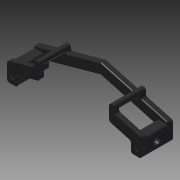
# Autodesk Inventor part: Solenoid Mount
Saved by Autodesk Inventor 2015 (Build 190159000, 159)
## iProperties
Created: 2016-09-23
Part Number: Solenoid Mount
Material: Generic
Document SubType Name: Modeling
Designer: James Yelland
Density: 1 g/cm^3
Appearance: Default
Author: James Yelland
Autodesk Inventor part; units mm, degrees
ref_plane "YZ Plane" through (0, 0, 0) normal (1, 0, 0) x (0, 1, 0)
ref_plane "XZ Plane" through (0, 0, 0) normal (0, 1, 0) x (-1, 0, 0)
ref_plane "XY Plane" through (0, 0, 0) normal (0, 0, 1) x (1, 0, 0)
sketch "Sketch1" plane through (0, 0, 0) normal (0, 1, 0) x (-1, 0, 0)
  line L0 (-54.0074, -78) -> (-54.0074, -71.5202)
  arc A0 (-52.5426, -69.5932) -> (-54.0074, -71.5202) centre (-52.0074, -71.5202) ccw
  arc A1 (-56.0074, -80) -> (-54.0074, -78) centre (-56.0074, -78) ccw
  line L1 (-54.0074, -78) -> (-54.0074, -71.5202)
  arc A2 (-52.5426, -69.5932) -> (-54.0074, -71.5202) centre (-52.0074, -71.5202) ccw
  arc A3 (-56.0074, -80) -> (-54.0074, -78) centre (-56.0074, -78) ccw
  line L2 (-54.0074, -78) -> (-54.0074, -71.5202)
  arc A4 (-52.5426, -69.5932) -> (-54.0074, -71.5202) centre (-52.0074, -71.5202) ccw
  arc A5 (-56.0074, -80) -> (-54.0074, -78) centre (-56.0074, -78) ccw
  line L3 (-62.0074, -80) -> (-56.0074, -80)
  line L4 (-64.0074, -78) -> (-64.0074, -64.2976)
  arc A6 (-62.5426, -62.3706) -> (-64.0074, -64.2976) centre (-62.0074, -64.2976) ccw
  arc A7 (-64.0074, -78) -> (-62.0074, -80) centre (-62.0074, -78) ccw
  line L5 (-52.5426, -69.5932) -> (-34.7368, -64.6478)
  line L6 (-33.272, -62.7207) -> (-33.272, -56.3381)
  line L7 (-33.272, -56.3381) -> (-33.272, -54)
  line L8 (-33.272, -54) -> (-33.272, -51)
  line L9 (-35.272, -49) -> (-36.272, -49)
  line L10 (-62.5426, -62.3706) -> (-39.7368, -56.0365)
  line L11 (-38.272, -54.1094) -> (-38.272, -51)
  arc A8 (-36.272, -49) -> (-38.272, -51) centre (-36.272, -51) ccw
  arc A9 (-33.272, -51) -> (-35.272, -49) centre (-35.272, -51) ccw
  arc A10 (-39.7368, -56.0365) -> (-38.272, -54.1094) centre (-40.272, -54.1094) ccw
  arc A11 (-34.7368, -64.6478) -> (-33.272, -62.7207) centre (-35.272, -62.7207) ccw
  line L12 (54.0074, -78) -> (54.0074, -71.5202)
  arc A12 (54.0074, -71.5202) -> (52.5426, -69.5932) centre (52.0074, -71.5202) ccw
  arc A13 (54.0074, -78) -> (56.0074, -80) centre (56.0074, -78) ccw
  line L13 (54.0074, -78) -> (54.0074, -71.5202)
  arc A14 (54.0074, -71.5202) -> (52.5426, -69.5932) centre (52.0074, -71.5202) ccw
  arc A15 (54.0074, -78) -> (56.0074, -80) centre (56.0074, -78) ccw
  line L14 (54.0074, -78) -> (54.0074, -71.5202)
  arc A16 (54.0074, -78) -> (56.0074, -80) centre (56.0074, -78) ccw
  arc A17 (54.0074, -71.5202) -> (52.5426, -69.5932) centre (52.0074, -71.5202) ccw
  line L15 (62.0074, -80) -> (56.0074, -80)
  line L16 (64.0074, -78) -> (64.0074, -64.2976)
  arc A18 (64.0074, -64.2976) -> (62.5426, -62.3706) centre (62.0074, -64.2976) ccw
  arc A19 (62.0074, -80) -> (64.0074, -78) centre (62.0074, -78) ccw
  line L17 (52.5426, -69.5932) -> (34.7368, -64.6478)
  line L18 (33.272, -62.7207) -> (33.272, -56.3381)
  line L19 (33.272, -56.3381) -> (33.272, -54)
  line L20 (33.272, -54) -> (33.272, -51)
  line L21 (35.272, -49) -> (36.272, -49)
  line L22 (62.5426, -62.3706) -> (39.7368, -56.0365)
  line L23 (38.272, -54.1094) -> (38.272, -51)
  arc A20 (38.272, -51) -> (36.272, -49) centre (36.272, -51) ccw
  arc A21 (35.272, -49) -> (33.272, -51) centre (35.272, -51) ccw
  arc A22 (38.272, -54.1094) -> (39.7368, -56.0365) centre (40.272, -54.1094) ccw
  arc A23 (33.272, -62.7207) -> (34.7368, -64.6478) centre (35.272, -62.7207) ccw
  point P0 (-33.272, -64.241)
  point P1 (-33.272, -49)
  point P2 (-38.272, -49)
  point P3 (33.272, -64.241)
  point P4 (33.272, -49)
  point P5 (38.272, -49)
  dimension "d11" = 2
  dimension "d29" = 20
  dimension "d30" = 5
  dimension "d31" = 5
  dimension "d32" = 2
  constraints: 48 end point, 48 point on circle, 24 centre point, 16 point on line, 13 tangent, 4 equal radius, 2 perpendicular, 1 vertical
  measures "d11" radius of A6
  measures "d29" distance of L5.start point (-33.272, -64.241)
  measures "d30" distance of L7.end point (-33.272, -49)
  measures "d31" distance of point (-33.272, -49) point (-38.272, -49)
  measures "d32" radius of A8
extrude "Extrusion1" add sketch "Sketch1" along normal blind 5
sketch "Sketch2" plane through (0, 5, 0) normal (0, 1, 0) x (1, 0, 0)
  line L0 (54.0074, 78) -> (54.0074, 71.5202) projected
  arc A0 (56.0074, 80) -> (54.0074, 78) centre (56.0074, 78) ccw projected
  line L1 (62.0074, 80) -> (56.0074, 80) projected
  arc A1 (64.0074, 78) -> (62.0074, 80) centre (62.0074, 78) ccw projected
  line L2 (64.0074, 64.2976) -> (64.0074, 78) projected
  line L3 (54.0074, 71.5202) -> (54.0074, 66.2976)
  line L4 (56.0074, 64.2976) -> (62.0074, 64.2976)
  line L5 (64.0074, 66.2976) -> (64.0074, 78)
  arc A2 (62.0074, 64.2976) -> (64.0074, 66.2976) centre (62.0074, 66.2976) ccw
  arc A3 (54.0074, 66.2976) -> (56.0074, 64.2976) centre (56.0074, 66.2976) ccw
  line L6 (0, 44.0707) -> (0, 74.7601)
  line L7 (-54.0074, 78) -> (-54.0074, 71.5202)
  arc A4 (-54.0074, 78) -> (-56.0074, 80) centre (-56.0074, 78) ccw
  line L8 (-62.0074, 80) -> (-56.0074, 80)
  arc A5 (-62.0074, 80) -> (-64.0074, 78) centre (-62.0074, 78) ccw
  line L9 (-64.0074, 64.2976) -> (-64.0074, 78)
  line L10 (-54.0074, 71.5202) -> (-54.0074, 66.2976)
  line L11 (-56.0074, 64.2976) -> (-62.0074, 64.2976)
  line L12 (-64.0074, 66.2976) -> (-64.0074, 78)
  arc A6 (-64.0074, 66.2976) -> (-62.0074, 64.2976) centre (-62.0074, 66.2976) ccw
  arc A7 (-56.0074, 64.2976) -> (-54.0074, 66.2976) centre (-56.0074, 66.2976) ccw
  line L13 (38.272, 51) -> (38.272, 54.1094) projected
  arc A8 (36.272, 49) -> (38.272, 51) centre (36.272, 51) ccw projected
  line L14 (35.272, 49) -> (36.272, 49) projected
  arc A9 (33.272, 51) -> (35.272, 49) centre (35.272, 51) ccw projected
  line L15 (33.272, 62.7207) -> (33.272, 51) projected
  line L16 (36.272, 49) -> (35.272, 49) projected
  line L17 (35.772, 49) -> (35.772, 54)
  line L18 (35.772, 54) -> (35.272, 54)
  line L19 (33.272, 51) -> (33.272, 62.7207) projected
  line L20 (35.772, 54) -> (36.272, 54)
  line L21 (38.272, 54.1094) -> (38.272, 51) projected
  line L22 (-38.272, 51) -> (-38.272, 52)
  arc A10 (-38.272, 51) -> (-36.272, 49) centre (-36.272, 51) ccw
  line L23 (-35.272, 49) -> (-36.272, 49)
  arc A11 (-35.272, 49) -> (-33.272, 51) centre (-35.272, 51) ccw
  line L24 (-33.272, 52) -> (-33.272, 51)
  line L25 (-36.272, 49) -> (-35.272, 49)
  line L26 (-35.772, 49) -> (-35.772, 54)
  line L27 (-35.772, 54) -> (-35.272, 54)
  line L28 (-33.272, 51) -> (-33.272, 62.7207)
  line L29 (-35.772, 54) -> (-36.272, 54)
  line L30 (-38.272, 54.1094) -> (-38.272, 51)
  line L31 (38.272, 52) -> (38.272, 51)
  line L32 (33.272, 52) -> (33.272, 51)
  arc A12 (-33.272, 52) -> (-35.272, 54) centre (-35.272, 52) ccw
  arc A13 (-36.272, 54) -> (-38.272, 52) centre (-36.272, 52) ccw
  arc A14 (38.272, 52) -> (36.272, 54) centre (36.272, 52) ccw
  arc A15 (35.272, 54) -> (33.272, 52) centre (35.272, 52) ccw
  point P0 (0, 0)
  point P1 (33.272, 54)
  point P2 (38.272, 54)
  point P3 (-33.272, 54)
  point P4 (-38.272, 54)
  dimension "d19" = 2
  dimension "d33" = 5
  dimension "d34" = 2
  constraints: 48 end point, 26 symmetric about line, 24 point on circle, 16 point on line, 12 centre point, 12 tangent, 4 equal radius, 4 vertical, 2 collinear, 2 perpendicular, 1 horizontal, 1 midpoint, 6 other
  measures "d19" radius of A2
  measures "d33" distance of L17.start L17.end
  measures "d34" radius of A12
extrude "Extrusion2" add sketch "Sketch2" along normal blind 20
sketch "Sketch3" plane through (0, 25, 0) normal (0, 1, 0) x (1, 0, 0)
  arc A0 (62.0074, 64.2976) -> (64.0074, 66.2976) centre (62.0074, 66.2976) ccw projected
  line L0 (62.0074, 64.2976) -> (56.0074, 64.2976) projected
  arc A1 (54.0074, 66.2976) -> (56.0074, 64.2976) centre (56.0074, 66.2976) ccw projected
  line L1 (54.0074, 66.2976) -> (54.0074, 71.5202) projected
  arc A2 (52.5426, 69.5932) -> (54.0074, 71.5202) centre (52.0074, 71.5202) ccw projected
  line L2 (52.5426, 69.5932) -> (34.7368, 64.6478) projected
  arc A3 (34.7368, 64.6478) -> (33.272, 62.7207) centre (35.272, 62.7207) ccw projected
  line L3 (33.272, 62.7207) -> (33.272, 52) projected
  arc A4 (35.272, 54) -> (33.272, 52) centre (35.272, 52) ccw projected
  line L4 (35.272, 54) -> (36.272, 54) projected
  arc A5 (38.272, 52) -> (36.272, 54) centre (36.272, 52) ccw projected
  line L5 (38.272, 52) -> (38.272, 54.1094) projected
  arc A6 (39.7368, 56.0365) -> (38.272, 54.1094) centre (40.272, 54.1094) ccw projected
  line L6 (39.7368, 56.0365) -> (62.5426, 62.3706) projected
  arc A7 (62.5426, 62.3706) -> (64.0074, 64.2976) centre (62.0074, 64.2976) ccw projected
  line L7 (64.0074, 64.2976) -> (64.0074, 66.2976) projected
  line L8 (54.0074, 78) -> (54.0074, 66.2976) projected
  arc A8 (54.0074, 66.2976) -> (56.0074, 64.2976) centre (56.0074, 66.2976) ccw projected
  line L9 (56.0074, 64.2976) -> (62.0074, 64.2976) projected
  arc A9 (62.0074, 64.2976) -> (64.0074, 66.2976) centre (62.0074, 66.2976) ccw projected
  line L10 (64.0074, 66.2976) -> (64.0074, 78) projected
  arc A10 (64.0074, 78) -> (62.0074, 80) centre (62.0074, 78) ccw projected
  line L11 (62.0074, 80) -> (56.0074, 80) projected
  arc A11 (56.0074, 80) -> (54.0074, 78) centre (56.0074, 78) ccw projected
  line L12 (38.272, 51) -> (38.272, 52) projected
  arc A12 (38.272, 52) -> (36.272, 54) centre (36.272, 52) ccw projected
  line L13 (36.272, 54) -> (35.272, 54) projected
  arc A13 (35.272, 54) -> (33.272, 52) centre (35.272, 52) ccw projected
  line L14 (33.272, 52) -> (33.272, 51) projected
  arc A14 (33.272, 51) -> (35.272, 49) centre (35.272, 51) ccw projected
  line L15 (35.272, 49) -> (36.272, 49) projected
  arc A15 (36.272, 49) -> (38.272, 51) centre (36.272, 51) ccw projected
  arc A16 (-33.272, 52) -> (-35.272, 54) centre (-35.272, 52) ccw projected
  line L16 (-33.272, 52) -> (-33.272, 62.7207) projected
  arc A17 (-33.272, 62.7207) -> (-34.7368, 64.6478) centre (-35.272, 62.7207) ccw projected
  line L17 (-34.7368, 64.6478) -> (-52.5426, 69.5932) projected
  arc A18 (-54.0074, 71.5202) -> (-52.5426, 69.5932) centre (-52.0074, 71.5202) ccw projected
  line L18 (-54.0074, 71.5202) -> (-54.0074, 66.2976) projected
  arc A19 (-56.0074, 64.2976) -> (-54.0074, 66.2976) centre (-56.0074, 66.2976) ccw projected
  line L19 (-56.0074, 64.2976) -> (-62.0074, 64.2976) projected
  arc A20 (-64.0074, 66.2976) -> (-62.0074, 64.2976) centre (-62.0074, 66.2976) ccw projected
  line L20 (-64.0074, 66.2976) -> (-64.0074, 64.2976) projected
  arc A21 (-64.0074, 64.2976) -> (-62.5426, 62.3706) centre (-62.0074, 64.2976) ccw projected
  line L21 (-62.5426, 62.3706) -> (-39.7368, 56.0365) projected
  arc A22 (-38.272, 54.1094) -> (-39.7368, 56.0365) centre (-40.272, 54.1094) ccw projected
  line L22 (-38.272, 54.1094) -> (-38.272, 52) projected
  arc A23 (-36.272, 54) -> (-38.272, 52) centre (-36.272, 52) ccw projected
  line L23 (-36.272, 54) -> (-35.272, 54) projected
  line L24 (-36.272, 49) -> (-35.272, 49) projected
  arc A24 (-35.272, 49) -> (-33.272, 51) centre (-35.272, 51) ccw projected
  line L25 (-33.272, 51) -> (-33.272, 52) projected
  arc A25 (-33.272, 52) -> (-35.272, 54) centre (-35.272, 52) ccw projected
  line L26 (-35.272, 54) -> (-36.272, 54) projected
  arc A26 (-36.272, 54) -> (-38.272, 52) centre (-36.272, 52) ccw projected
  line L27 (-38.272, 52) -> (-38.272, 51) projected
  arc A27 (-38.272, 51) -> (-36.272, 49) centre (-36.272, 51) ccw projected
  line L28 (-54.0074, 66.2976) -> (-54.0074, 78) projected
  arc A28 (-54.0074, 78) -> (-56.0074, 80) centre (-56.0074, 78) ccw projected
  line L29 (-56.0074, 80) -> (-62.0074, 80) projected
  arc A29 (-62.0074, 80) -> (-64.0074, 78) centre (-62.0074, 78) ccw projected
  line L30 (-64.0074, 78) -> (-64.0074, 66.2976) projected
  arc A30 (-64.0074, 66.2976) -> (-62.0074, 64.2976) centre (-62.0074, 66.2976) ccw projected
  line L31 (-62.0074, 64.2976) -> (-56.0074, 64.2976) projected
  arc A31 (-56.0074, 64.2976) -> (-54.0074, 66.2976) centre (-56.0074, 66.2976) ccw projected
  line L32 (52.5426, 69.5932) -> (0.5352, 55.1487)
  line L33 (34.7368, 64.6478) -> (52.5426, 69.5932) projected
  line L34 (-0.5352, 55.1487) -> (-34.7368, 64.6478)
  line L35 (0.5352, 45.1487) -> (30.7368, 53.5368)
  line L36 (-0.5352, 45.1487) -> (-30.7368, 53.5368)
  arc A32 (-0.5352, 45.1487) -> (0.5352, 45.1487) centre (0, 47.0757) ccw
  arc A33 (-0.5352, 55.1487) -> (0.5352, 55.1487) centre (0, 57.0757) ccw
  line L37 (33.272, 51) -> (33.272, 62.7207) projected
  line L38 (33.272, 51.6098) -> (33.272, 51)
  arc A34 (33.272, 51.6098) -> (30.7368, 53.5368) centre (31.272, 51.6098) ccw
  line L39 (-33.272, 51) -> (-33.272, 51.6098)
  line L40 (-33.272, 52) -> (-33.272, 62.7207) projected
  arc A35 (-30.7368, 53.5368) -> (-33.272, 51.6098) centre (-31.272, 51.6098) ccw
  line L41 (-34.7368, 64.6478) -> (-52.5426, 69.5932)
  arc A36 (-54.0074, 71.5202) -> (-52.5426, 69.5932) centre (-52.0074, 71.5202) ccw projected
  arc A37 (-54.0074, 71.5202) -> (-52.5426, 69.5932) centre (-52.0074, 71.5202) ccw
  arc A38 (-54.0074, 78) -> (-56.0074, 80) centre (-56.0074, 78) ccw
  arc A39 (-62.0074, 80) -> (-64.0074, 78) centre (-62.0074, 78) ccw
  arc A40 (-64.0074, 64.2976) -> (-62.5426, 62.3706) centre (-62.0074, 64.2976) ccw
  arc A41 (-38.272, 54.1094) -> (-39.7368, 56.0365) centre (-40.272, 54.1094) ccw
  arc A42 (-38.272, 51) -> (-36.272, 49) centre (-36.272, 51) ccw
  arc A43 (-35.272, 49) -> (-33.272, 51) centre (-35.272, 51) ccw
  arc A44 (52.5426, 69.5932) -> (54.0074, 71.5202) centre (52.0074, 71.5202) ccw
  arc A45 (56.0074, 80) -> (54.0074, 78) centre (56.0074, 78) ccw
  arc A46 (64.0074, 78) -> (62.0074, 80) centre (62.0074, 78) ccw
  arc A47 (62.5426, 62.3706) -> (64.0074, 64.2976) centre (62.0074, 64.2976) ccw
  arc A48 (39.7368, 56.0365) -> (38.272, 54.1094) centre (40.272, 54.1094) ccw
  arc A49 (36.272, 49) -> (38.272, 51) centre (36.272, 51) ccw
  arc A50 (33.272, 51) -> (35.272, 49) centre (35.272, 51) ccw
  line L42 (38.272, 54.1094) -> (38.272, 51)
  line L43 (36.272, 49) -> (35.272, 49)
  line L44 (39.7368, 56.0365) -> (62.5426, 62.3706)
  line L45 (64.0074, 64.2976) -> (64.0074, 78)
  line L46 (62.0074, 80) -> (56.0074, 80)
  line L47 (54.0074, 78) -> (54.0074, 71.5202)
  arc A51 (52.5426, 69.5932) -> (54.0074, 71.5202) centre (52.0074, 71.5202) ccw projected
  arc A52 (56.0074, 80) -> (54.0074, 78) centre (56.0074, 78) ccw projected
  line L48 (-54.0074, 71.5202) -> (-54.0074, 78)
  arc A53 (-54.0074, 78) -> (-56.0074, 80) centre (-56.0074, 78) ccw projected
  line L49 (-56.0074, 80) -> (-62.0074, 80)
  line L50 (-62.0074, 80) -> (-56.0074, 80) projected
  line L51 (-64.0074, 78) -> (-64.0074, 64.2976)
  line L52 (-62.5426, 62.3706) -> (-39.7368, 56.0365)
  line L53 (-62.5426, 62.3706) -> (-39.7368, 56.0365) projected
  line L54 (-38.272, 54.1094) -> (-38.272, 51)
  line L55 (-36.272, 49) -> (-35.272, 49)
  arc A54 (-38.272, 51) -> (-36.272, 49) centre (-36.272, 51) ccw projected
  point P0 (0, 0)
  point P1 (33.272, 54.241)
  point P2 (-33.272, 54.241)
  dimension "d61" = 2
  dimension "d62" = 2
  dimension "d63" = 2
  dimension "d64" = 2
  constraints: 38 end point, 36 point on circle, 18 centre point, 14 coincident, 13 tangent, 8 point on line, 7 collinear, 6 vertical, 2 horizontal
  measures "d61" radius of A32
  measures "d62" radius of A33
  measures "d63" radius of A34
  measures "d64" radius of A35
extrude "Extrusion3" add sketch "Sketch3" along normal blind 5
sketch "Sketch4" plane through (0, 30, 0) normal (0, 1, 0) x (1, 0, 0)
  line L0 (54.0074, 71.5202) -> (54.0074, 78) projected
  line L1 (54.0074, 74.7601) -> (59.2474, 74.7601)
  circle A0 centre (59.2474, 74.7601) radius 1.6
  line L2 (-54.0074, 78) -> (-54.0074, 71.5202) projected
  line L3 (-54.0074, 74.7601) -> (-59.2474, 74.7601)
  circle A1 centre (-59.2474, 74.7601) radius 1.6
  point P0 (0, 0)
  dimension "d37" = 5.24
  dimension "d38" = 3.2
  dimension "d39" = 5.24
  dimension "d40" = 3.2
  constraints: 4 end point, 2 centre point, 2 coincident, 2 horizontal, 2 midpoint
  measures "d37" distance of L1.start L1.end
  measures "d38" diameter of A0
  measures "d39" distance of L3.start L3.end
  measures "d40" diameter of A1
extrude "Extrusion4" cut sketch "Sketch4" against normal through all
fillet "Fillet1" radius 1 18 edges at (63.5996, 5, -63.0873) (64.0074, 5, -65.2976) (38.6798, 5, -55.3197) (38.272, 5, -53.0547) (51.1397, 5, -59.2035) (33.272, 5, -57.3604) (43.6397, 5, -67.1205) (53.5996, 5, -70.3099) (33.6798, 5, -63.931) (-53.5996, 5, -70.3099) (-33.6798, 5, -63.931) (-33.272, 5, -57.3604) (-43.6397, 5, -67.1205) (-38.272, 5, -53.0547) (-51.1397, 5, -59.2035) (-63.5996, 5, -63.0873) (-64.0074, 5, -65.2976) (-38.6798, 5, -55.3197)
fillet "Fillet2" radius 1 10 edges at (53.5996, 25, -70.3099) (64.0074, 25, -65.2976) (51.1397, 25, -59.2035) (-26.5389, 25, -62.3709) (-53.5996, 25, -70.3099) (-38.6798, 25, -55.3197) (-38.272, 25, -53.0547) (-63.5996, 25, -63.0873) (-64.0074, 25, -65.2976) (-51.1397, 25, -59.2035)
sketch "Sketch5" plane through (54.0074, 0, -78) normal (-1, 0, 0) x (0, 0, 1)
  line L0 (0, 30) -> (6.4798, 30) projected
  line L1 (6.4798, 30) -> (5.4798, 30)
  line L2 (5.4798, 30) -> (5.4798, 15)
  circle A0 centre (5.4798, 15) radius 3.25
  point P0 (78, 0)
  dimension "d48" = 1
  dimension "d49" = 15
  dimension "d50" = 6.5
  constraints: 4 end point, 1 centre point, 1 coincident, 1 perpendicular, 1 point on line
  measures "d48" distance of L0.end L1.end
  measures "d49" distance of L1.end L2.end
  measures "d50" diameter of A0
extrude "Extrusion5" cut sketch "Sketch5" against normal through all
sketch "Sketch6" plane through (54.0074, 0, -78) normal (-1, 0, 0) x (0, 0, 1)
  circle A0 centre (5.4798, 15) radius 3.25 projected
  circle A1 centre (5.4798, 15) radius 5
  point P0 (78, 0)
  dimension "d53" = 10
  constraints: 1 centre point, 1 coincident
  measures "d53" diameter of A1
extrude "Extrusion6" add sketch "Sketch6" along normal blind 2
chamfer "Chamfer1" distance 0.75 distance2 2 1 edges at (52.0074, 15, -77.5202) measured on face at (52.0074, 15, -77.0202)
fillet "Fillet3" radius 1 5 edges at (0, 25, -45.0757) (15.636, 25, -49.3427) (32.4823, 25, -53.202) (-32.4823, 25, -53.202) (-15.636, 25, -49.3427)
body "Solid1"
